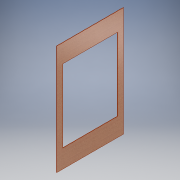
# Autodesk Inventor part: Frontal
Saved by Autodesk Inventor 2017 (Build 210142000, 142)
## iProperties
Created: 2017-10-10
Part Number: Frontal
Material: Wood (Oak)
Document SubType Name: Modeling
Designer: Felipe
Density: 0.76 g/cm^3
Appearance: White Oak - Natural Medium Gloss
Author: Felipe
Autodesk Inventor part; units mm, degrees
ref_plane "YZ Plane" through (0, 0, 0) normal (1, 0, 0) x (0, 1, 0)
ref_plane "XZ Plane" through (0, 0, 0) normal (0, 1, 0) x (-1, 0, 0)
ref_plane "XY Plane" through (0, 0, 0) normal (0, 0, 1) x (1, 0, 0)
sketch "Sketch1" plane through (0, 0, 0) normal (1, 0, 0) x (0, 1, 0)
  line L0 (0, 0) -> (549, 0)
  line L1 (549, 0) -> (549, -900)
  line L2 (549, -900) -> (0, -900)
  line L3 (0, -900) -> (0, 0)
  line L4 (499.5, -150) -> (49.5, -150)
  line L5 (49.5, -150) -> (49.5, -750)
  line L6 (49.5, -750) -> (499.5, -750)
  line L7 (499.5, -750) -> (499.5, -150)
  dimension "d0" = 549
  dimension "d1" = 900
  dimension "d2" = 600
  dimension "d3" = 450
  dimension "d4" = 49.5
  dimension "d5" = 150
  constraints: 16 end point, 4 parallel, 2 horizontal, 2 perpendicular
  measures "d0" distance of L0.start L0.end
  measures "d1" distance of L2.end L0.start
  measures "d2" distance of L6.end L4.start
  measures "d3" distance of L4.start L4.end
  measures "d4" distance between parallel lines of L1 L7
  measures "d5" distance between parallel lines of L2 L6
extrude "Extrusion1" add sketch "Sketch1" along normal blind 3
body "Solid1"
